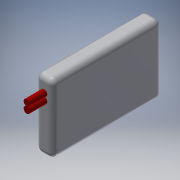
# Autodesk Inventor part: adafruit 500mAh battery
Saved by Autodesk Inventor 2016 (Build 200138000, 138)
## iProperties
Created: 2015-12-16
Part Number: adafruit 500mAh battery
Material: Generic
Document SubType Name: Modeling
Designer: benja
Density: 1 g/cm^3
Appearance: Default
Author: benja
Autodesk Inventor part; units mm, degrees
ref_plane "YZ Plane" through (0, 0, 0) normal (1, 0, 0) x (0, 1, 0)
ref_plane "XZ Plane" through (0, 0, 0) normal (0, 1, 0) x (-1, 0, 0)
ref_plane "XY Plane" through (0, 0, 0) normal (0, 0, 1) x (1, 0, 0)
sketch "Sketch1" plane through (0, 0, 0) normal (1, 0, 0) x (0, 1, 0)
  line L0 (0, 0) -> (20, 0)
  line L1 (20, 0) -> (20, 31.4)
  line L2 (20, 31.4) -> (0, 31.4)
  line L3 (0, 31.4) -> (0, 0)
  dimension "d0" = 20
  dimension "d1" = 31.4
  constraints: 8 end point, 2 parallel, 1 horizontal, 1 perpendicular
  measures "d0" distance of L2.end L1.end
  measures "d1" distance of L1.end L0.end
extrude "Extrusion1" add sketch "Sketch1" along normal blind 5
fillet "Fillet1" radius 1.5875 12 edges at (0, 0, 15.7) (2.5, 0, 0) (5, 0, 15.7) (2.5, 0, 31.4) (0, 10, 31.4) (5, 10, 31.4) (2.5, 20, 31.4) (0, 20, 15.7) (5, 20, 15.7) (2.5, 20, 0) (0, 10, 0) (5, 10, 0)
sketch "Sketch2" plane through (1.5875, 1.5875, 31.4) normal (0, 0, 1) x (1, 0, 0)
  line L0 (0, 0) -> (0, 16.825) projected
  line L1 (1.825, 0) -> (0, 0) projected
  line L2 (1.825, 16.825) -> (1.825, 0) projected
  circle A0 centre (0.9125, 14.325) radius 0.9125
  circle A1 centre (0.9125, 12.5) radius 0.9125
  point P0 (-1.5875, -1.5875)
  dimension "d5" = 12.5
  constraints: 4 tangent, 2 centre point, 1 equal radius
  measures "d5" distance from line of L1 A1.centre
extrude "Extrusion2" add sketch "Sketch2" along normal blind 5 contours A1 | A0
body "Solid1"
